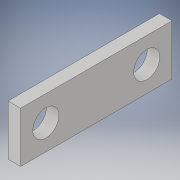
# Autodesk Inventor part: clampPlate
Saved by Autodesk Inventor 2019 (Build 230136000, 136)
## iProperties
Created: 2019-02-03
Part Number: clampPlate
Material: Generic
Document SubType Name: Modeling
Designer: james
Density: 1 g/cm^3
Appearance: Default
Author: james
Autodesk Inventor part; units mm, degrees
ref_plane "YZ Plane" through (0, 0, 0) normal (1, 0, 0) x (0, 1, 0)
ref_plane "XZ Plane" through (0, 0, 0) normal (0, 1, 0) x (-1, 0, 0)
ref_plane "XY Plane" through (0, 0, 0) normal (0, 0, 1) x (1, 0, 0)
sketch "Sketch1" plane through (0, 0, 0) normal (1, 0, 0) x (0, 1, 0)
  line L0 (4.3974, 6.5718) -> (-1.9526, 6.5718)
  line L1 (-1.9526, 6.5718) -> (-1.9526, -12.4782)
  line L2 (-1.9526, -12.4782) -> (4.3974, -12.4782)
  line L3 (4.3974, -12.4782) -> (4.3974, 6.5718)
  point P0 (0, 0)
  dimension "d0" = 19.05
  dimension "d1" = 6.35
  constraints: 8 end point, 2 parallel, 1 horizontal, 1 perpendicular
  measures "d0" distance of L2.end L0.start
  measures "d1" distance of L0.start L0.end
extrude "Extrusion1" add sketch "Sketch1" along normal blind 1.5875
sketch "Sketch2" plane through (1.5875, 0, 0) normal (1, 0, 0) x (0, 0, -1)
  line L0 (12.4782, 4.3974) -> (-6.5718, 4.3974) projected
  line L1 (-6.5718, 4.3974) -> (-6.5718, -1.9526) projected
  line L2 (12.4782, -1.9526) -> (12.4782, 4.3974) projected
  point P0 (0, 0)
  point P1 (-3.3968, 1.2224)
  point P2 (9.3032, 1.2224)
  dimension "d4" = 3.175
  dimension "d5" = 3.175
  dimension "d6" = 3.175
  measures "d4" distance from line of L0 point (-3.397, 1.222)
  measures "d5" distance from line of L1 point (-3.397, 1.222)
  measures "d6" distance from line of L2 point (9.303, 1.222)
hole "Hole1" at (1.5875, 1.2224, 3.3968) at (1.5875, 1.2224, -9.3032) direction (-1, 0, 0) diameter 3.302 depth 25.4 tip angle 118.188
body "Solid1"
